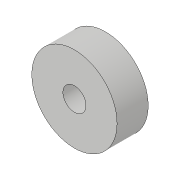
# Autodesk Inventor part: Ball Bearing
Saved by Autodesk Inventor 2018.3 (Build 223284000, 284)
## iProperties
Created: 2019-03-08
Part Number: Ball Bearing
Material: Generic
Document SubType Name: Modeling
Designer: aye06091
Mass: 1.41514 g
Surface Area: 8.88316 cm^2
Volume: 1.41514 cm^3
Density: 1 g/cm^3
Appearance: Default
Author: aye06091
Autodesk Inventor part; units mm, degrees
ref_plane "YZ Plane" through (0, 0, 0) normal (1, 0, 0) x (0, 1, 0)
ref_plane "XZ Plane" through (0, 0, 0) normal (0, 1, 0) x (-1, 0, 0)
ref_plane "XY Plane" through (0, 0, 0) normal (0, 0, 1) x (1, 0, 0)
sketch "Sketch1" plane through (0, 0, 0) normal (0, 0, 1) x (1, 0, 0)
  circle A0 centre (0, 0) radius 2.3622
  circle A1 centre (0, 0) radius 8.7313
  dimension "d0" = 4.7244
  dimension "d1" = 17.4625
  constraints: 2 centre point, 2 coincident
  measures "d0" diameter of A0
  measures "d1" diameter of A1
extrude "Extrusion1" add sketch "Sketch1" along normal blind 6.3754
body "Solid1"
